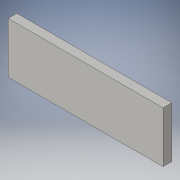
# Autodesk Inventor part: mcdave breadboard
Saved by Autodesk Inventor 2016 (Build 200138000, 138)
## iProperties
Created: 2016-10-04
Part Number: mcdave breadboard
Material: Generic
Document SubType Name: Modeling
Designer: ClenoR
Density: 1 g/cm^3
Appearance: Default
Author: ClenoR
Autodesk Inventor part; units mm, degrees
ref_plane "YZ Plane" through (0, 0, 0) normal (1, 0, 0) x (0, 1, 0)
ref_plane "XZ Plane" through (0, 0, 0) normal (0, 1, 0) x (-1, 0, 0)
ref_plane "XY Plane" through (0, 0, 0) normal (0, 0, 1) x (1, 0, 0)
sketch "Sketch1" plane through (0, 0, 0) normal (0, 0, 1) x (1, 0, 0)
  line L0 (-121.3282, 21.7984) -> (43.7718, 21.7984)
  line L1 (43.7718, 21.7984) -> (43.7718, -32.5576)
  line L2 (43.7718, -32.5576) -> (-121.3282, -32.5576)
  line L3 (-121.3282, -32.5576) -> (-121.3282, 21.7984)
  point P0 (0, 0)
  dimension "d0" = 54.356
  dimension "d1" = 165.1
  constraints: 8 end point, 2 parallel, 1 horizontal, 1 perpendicular
  measures "d0" distance of L0.end L1.end
  measures "d1" distance of L0.start L0.end
extrude "Extrusion1" add sketch "Sketch1" along normal blind 9.3726
body "Solid1"
